Autodesk Inventor part; units mm, degrees
(part 4 of 5)
  line L2655 (4.6359, 9.411) -> (5.6545, 8.2226)
  line L2656 (5.6545, 8.2226) -> (6.2587, 6.9004)
  line L2657 (6.2587, 6.9004) -> (6.4483, 5.4445)
  line L2658 (6.4483, 5.4445) -> (6.2234, 3.8548)
  line L2659 (6.2234, 3.8548) -> (4.7682, 3.4579)
  line L2660 (4.7682, 3.4579) -> (2.8432, 1.5333)
  line L2661 (2.8432, 1.5333) -> (1.064, -0.5108)
  line L2662 (1.064, -0.5108) -> (0.4492, -0.9828)
  line L2663 (0.4492, -0.9828) -> (-0.1305, -1.1181)
  line L2664 (-0.1305, -1.1181) -> (-0.6753, -0.9167)
  line L2665 (-0.6753, -0.9167) -> (-1.185, -0.3785)
  line L2666 (-1.185, -0.3785) -> (-1.2307, 0.9395)
  line L2667 (-1.2307, 0.9395) -> (-1.4443, 2.2167)
  line L2668 (-1.4443, 2.2167) -> (-1.826, 3.453)
  line L2669 (-1.826, 3.453) -> (-2.3756, 4.6485)
  line L2670 (-2.3756, 4.6485) -> (-2.111, 5.31)
  line L2671 (-2.111, 5.31) -> (-2.6223, 7.4795)
  line L2672 (-2.6223, 7.4795) -> (-2.6402, 9.6756)
  line L2673 (-2.6402, 9.6756) -> (-2.036, 11.356)
  line L2674 (-2.036, 11.356) -> (-1.7141, 13.1152)
  line L2675 (-1.7141, 13.1152) -> (0.0057, 15.761)
  line L2676 (-93.9213, 13.6444) -> (-93.19, 13.4597)
  line L2677 (-93.19, 13.4597) -> (-92.7037, 13.0895)
  line L2678 (-92.7037, 13.0895) -> (-92.4624, 12.5337)
  line L2679 (-92.4624, 12.5337) -> (-92.4661, 11.7923)
  line L2680 (-92.4661, 11.7923) -> (-92.7187, 10.8772)
  line L2681 (-92.7187, 10.8772) -> (-93.1336, 10.065)
  line L2682 (-93.1336, 10.065) -> (-93.7109, 9.3558)
  line L2683 (-93.7109, 9.3558) -> (-94.4505, 8.7496)
  line L2684 (-94.4505, 8.7496) -> (-95.0008, 8.6392)
  line L2685 (-95.0008, 8.6392) -> (-95.4488, 8.7347)
  line L2686 (-95.4488, 8.7347) -> (-95.7945, 9.0361)
  line L2687 (-95.7945, 9.0361) -> (-96.038, 9.5433)
  line L2688 (-96.038, 9.5433) -> (-93.9213, 13.6444)
  line L2689 (7.9432, 12.586) -> (8.4146, 12.3444)
  line L2690 (8.4146, 12.3444) -> (8.7702, 11.9992)
  line L2691 (8.7702, 11.9992) -> (9.1338, 10.9985)
  line L2692 (9.1338, 10.9985) -> (9.2661, 10.2048)
  line L2693 (9.2661, 10.2048) -> (9.1338, 9.411)
  line L2694 (9.1338, 9.411) -> (8.6046, 9.1465)
  line L2695 (8.6046, 9.1465) -> (8.0754, 9.411)
  line L2696 (8.0754, 9.411) -> (7.6146, 10.2012)
  line L2697 (7.6146, 10.2012) -> (7.4389, 10.9938)
  line L2698 (7.4389, 10.9938) -> (7.5484, 11.7887)
  line L2699 (7.5484, 11.7887) -> (7.9432, 12.586)
  line L2700 (-111.6484, -1.966) -> (-115.0879, -1.966)
  line L2701 (-115.0879, -1.966) -> (-115.6171, 0.1506)
  line L2702 (-115.6171, 0.1506) -> (-115.0879, 1.4735)
  line L2703 (-115.0879, 1.4735) -> (-115.2202, 6.236)
  line L2704 (-115.2202, 6.236) -> (-116.014, 7.5589)
  line L2705 (-116.014, 7.5589) -> (-116.4749, 9.612)
  line L2706 (-116.4749, 9.612) -> (-117.2046, 11.5277)
  line L2707 (-117.2046, 11.5277) -> (-116.4109, 11.3954)
  line L2708 (-116.4109, 11.3954) -> (-115.3525, 9.8079)
  line L2709 (-115.3525, 9.8079) -> (-114.4461, 9.4186)
  line L2710 (-114.4461, 9.4186) -> (-113.6327, 8.8819)
  line L2711 (-113.6327, 8.8819) -> (-113.3653, 7.6773)
  line L2712 (-113.3653, 7.6773) -> (-112.5744, 6.7652)
  line L2713 (-112.5744, 6.7652) -> (-112.1109, 4.5977)
  line L2714 (-112.1109, 4.5977) -> (-111.802, 2.42)
  line L2715 (-111.802, 2.42) -> (-111.6479, 0.2321)
  line L2716 (-111.6479, 0.2321) -> (-111.6484, -1.966)
  line L2717 (-58.9963, 11.5277) -> (-57.2942, 11.4904)
  line L2718 (-57.2942, 11.4904) -> (-55.6891, 10.9985)
  line L2719 (-55.6891, 10.9985) -> (-55.6883, 9.9418)
  line L2720 (-55.6883, 9.9418) -> (-55.8865, 8.9502)
  line L2721 (-55.8865, 8.9502) -> (-56.2836, 8.0236)
  line L2722 (-56.2836, 8.0236) -> (-56.8797, 7.1621)
  line L2723 (-56.8797, 7.1621) -> (-57.6002, 7.1375)
  line L2724 (-57.6002, 7.1375) -> (-58.2026, 7.5589)
  line L2725 (-58.2026, 7.5589) -> (-58.5305, 7.2355)
  line L2726 (-58.5305, 7.2355) -> (-58.8823, 7.0837)
  line L2727 (-58.8823, 7.0837) -> (-59.258, 7.1033)
  line L2728 (-59.258, 7.1033) -> (-59.6578, 7.2944)
  line L2729 (-59.6578, 7.2944) -> (-59.1319, 9.3325)
  line L2730 (-59.1319, 9.3325) -> (-58.9963, 11.5277)
  line L2731 (-138.1067, 11.2631) -> (-136.4181, 10.9747)
  line L2732 (-136.4181, 10.9747) -> (-134.9317, 10.2048)
  line L2733 (-134.9317, 10.2048) -> (-136.3974, 8.9662)
  line L2734 (-136.3974, 8.9662) -> (-138.1067, 8.0881)
  line L2735 (-138.1067, 8.0881) -> (-138.1067, 11.2631)
  line L2736 (-20.6318, 9.6756) -> (-19.4196, 9.5125)
  line L2737 (-19.4196, 9.5125) -> (-18.2506, 9.1464)
  line L2738 (-18.2506, 9.1464) -> (-18.2905, 7.3941)
  line L2739 (-18.2905, 7.3941) -> (-18.912, 5.7069)
  line L2740 (-18.912, 5.7069) -> (-19.7058, 5.1777)
  line L2741 (-19.7058, 5.1777) -> (-21.2933, 7.2944)
  line L2742 (-21.2933, 7.2944) -> (-21.4336, 8.0061)
  line L2743 (-21.4336, 8.0061) -> (-21.3701, 8.6402)
  line L2744 (-21.3701, 8.6402) -> (-21.1028, 9.1967)
  line L2745 (-21.1028, 9.1967) -> (-20.6318, 9.6756)
  line L2746 (0.7994, 9.1464) -> (1.3625, 9.1738)
  line L2747 (1.3625, 9.1738) -> (1.8148, 9.0286)
  line L2748 (1.8148, 9.0286) -> (2.1563, 8.7108)
  line L2749 (2.1563, 8.7108) -> (2.3869, 8.2204)
  line L2750 (2.3869, 8.2204) -> (2.2879, 7.5492)
  line L2751 (2.2879, 7.5492) -> (2.0565, 7.2152)
  line L2752 (2.0565, 7.2152) -> (1.6926, 7.2184)
  line L2753 (1.6926, 7.2184) -> (1.1963, 7.5589)
  line L2754 (1.1963, 7.5589) -> (0.8732, 8.3219)
  line L2755 (0.8732, 8.3219) -> (0.7994, 9.1464)
  line L2756 (-103.9755, 8.6173) -> (-103.4906, 8.3478)
  line L2757 (-103.4906, 8.3478) -> (-103.2849, 8.0376)
  line L2758 (-103.2849, 8.0376) -> (-103.3583, 7.6864)
  line L2759 (-103.3583, 7.6864) -> (-103.7109, 7.2944)
  line L2760 (-103.7109, 7.2944) -> (-103.9659, 7.9317)
  line L2761 (-103.9659, 7.9317) -> (-103.9755, 8.6173)
  line L2762 (-84.1317, 8.3527) -> (-83.4703, 7.8235)
  line L2763 (-83.4703, 7.8235) -> (-83.341, 6.7532)
  line L2764 (-83.341, 6.7532) -> (-83.6026, 5.7069)
  line L2765 (-83.6026, 5.7069) -> (-84.2653, 6.2709)
  line L2766 (-84.2653, 6.2709) -> (-84.5745, 6.8999)
  line L2767 (-84.5745, 6.8999) -> (-84.53, 7.5938)
  line L2768 (-84.53, 7.5938) -> (-84.1317, 8.3527)
  line L2769 (-29.0985, 7.0298) -> (-28.4104, 6.7294)
  line L2770 (-28.4104, 6.7294) -> (-27.9606, 6.2985)
  line L2771 (-27.9606, 6.2985) -> (-27.749, 5.7372)
  line L2772 (-27.749, 5.7372) -> (-27.7756, 5.0454)
  line L2773 (-27.7756, 5.0454) -> (-28.7088, 5.1098)
  line L2774 (-28.7088, 5.1098) -> (-29.2403, 5.4619)
  line L2775 (-29.2403, 5.4619) -> (-29.3702, 6.1019)
  line L2776 (-29.3702, 6.1019) -> (-29.0985, 7.0298)
  line L2777 (-91.5401, -1.966) -> (-93.3921, -1.966)
  line L2778 (-93.3921, -1.966) -> (-93.2044, -0.9504)
  line L2779 (-93.2044, -0.9504) -> (-92.863, 0.0183)
  line L2780 (-92.863, 0.0183) -> (-93.6713, 0.7264)
  line L2781 (-93.6713, 0.7264) -> (-94.4699, 0.9404)
  line L2782 (-94.4699, 0.9404) -> (-95.2588, 0.6603)
  line L2783 (-95.2588, 0.6603) -> (-96.038, -0.114)
  line L2784 (-96.038, -0.114) -> (-96.5671, -1.966)
  line L2785 (-96.5671, -1.966) -> (-98.9484, -1.966)
  line L2786 (-98.9484, -1.966) -> (-99.3742, -0.3196)
  line L2787 (-99.3742, -0.3196) -> (-100.139, 1.209)
  line L2788 (-100.139, 1.209) -> (-100.8005, 4.6485)
  line L2789 (-100.8005, 4.6485) -> (-100.6806, 5.3724)
  line L2790 (-100.6806, 5.3724) -> (-100.2713, 5.9714)
  line L2791 (-100.2713, 5.9714) -> (-98.1546, 6.7652)
  line L2792 (-98.1546, 6.7652) -> (-97.4932, 6.236)
  line L2793 (-97.4932, 6.236) -> (-97.2526, 5.4664)
  line L2794 (-97.2526, 5.4664) -> (-96.8637, 4.813)
  line L2795 (-96.8637, 4.813) -> (-96.3265, 4.2758)
  line L2796 (-96.3265, 4.2758) -> (-95.6411, 3.8548)
  line L2797 (-95.6411, 3.8548) -> (-95.4814, 3.1188)
  line L2798 (-95.4814, 3.1188) -> (-95.1856, 2.4766)
  line L2799 (-95.1856, 2.4766) -> (-94.7538, 1.9282)
  line L2800 (-94.7538, 1.9282) -> (-94.1859, 1.4735)
  line L2801 (-94.1859, 1.4735) -> (-93.4772, 1.7841)
  line L2802 (-93.4772, 1.7841) -> (-92.863, 2.2673)
  line L2803 (-92.863, 2.2673) -> (-91.9757, 0.2264)
  line L2804 (-91.9757, 0.2264) -> (-91.5401, -1.966)
  line L2805 (16.1452, 6.7652) -> (16.5067, 6.4551)
  line L2806 (16.5067, 6.4551) -> (16.6051, 6.1313)
  line L2807 (16.6051, 6.1313) -> (16.4406, 5.7937)
  line L2808 (16.4406, 5.7937) -> (16.0129, 5.4423)
  line L2809 (16.0129, 5.4423) -> (15.753, 5.7888)
  line L2810 (15.753, 5.7888) -> (15.6885, 6.1249)
  line L2811 (15.6885, 6.1249) -> (15.8192, 6.4503)
  line L2812 (15.8192, 6.4503) -> (16.1452, 6.7652)
  line L2813 (-34.9193, 6.236) -> (-33.5964, 6.236)
  line L2814 (-33.5964, 6.236) -> (-33.6618, 5.6624)
  line L2815 (-33.6618, 5.6624) -> (-33.904, 5.2947)
  line L2816 (-33.904, 5.2947) -> (-34.3232, 5.1331)
  line L2817 (-34.3232, 5.1331) -> (-34.9193, 5.1777)
  line L2818 (-34.9193, 5.1777) -> (-34.9193, 6.236)
  line L2819 (-109.2671, -1.966) -> (-110.0609, -1.966)
  line L2820 (-110.0609, -1.966) -> (-110.4665, 1.5949)
  line L2821 (-110.4665, 1.5949) -> (-110.4577, 5.1777)
  line L2822 (-110.4577, 5.1777) -> (-109.9354, 5.2372)
  line L2823 (-109.9354, 5.2372) -> (-109.5628, 5.0806)
  line L2824 (-109.5628, 5.0806) -> (-109.34, 4.708)
  line L2825 (-109.34, 4.708) -> (-109.2671, 4.1194)
  line L2826 (-109.2671, 4.1194) -> (-109.5755, 2.8028)
  line L2827 (-109.5755, 2.8028) -> (-109.664, 1.4735)
  line L2828 (-109.664, 1.4735) -> (-108.4734, -0.114)
  line L2829 (-108.4734, -0.114) -> (-109.2671, -1.966)
  line L2830 (-138.1067, 4.9131) -> (-137.3778, 4.2285)
  line L2831 (-137.3778, 4.2285) -> (-137.1349, 3.5593)
  line L2832 (-137.1349, 3.5593) -> (-137.3778, 2.9056)
  line L2833 (-137.3778, 2.9056) -> (-138.1067, 2.2673)
  line L2834 (-138.1067, 2.2673) -> (-138.1067, 4.9131)
  line L2835 (-51.588, -1.966) -> (-53.1755, -1.966)
  line L2836 (-53.1755, -1.966) -> (-52.9109, -0.2463)
  line L2837 (-52.9109, -0.2463) -> (-53.9693, 3.8548)
  line L2838 (-53.9693, 3.8548) -> (-53.3078, 4.6485)
  line L2839 (-53.3078, 4.6485) -> (-50.7943, 3.9871)
  line L2840 (-50.7943, 3.9871) -> (-50.3295, 2.8687)
  line L2841 (-50.3295, 2.8687) -> (-50.2651, 1.7381)
  line L2842 (-50.2651, 1.7381) -> (-50.5773, 2.1062)
  line L2843 (-50.5773, 2.1062) -> (-50.8799, 2.2289)
  line L2844 (-50.8799, 2.2289) -> (-51.1727, 2.1062)
  line L2845 (-51.1727, 2.1062) -> (-51.4557, 1.7381)
  line L2846 (-51.4557, 1.7381) -> (-51.3882, -0.1189)
  line L2847 (-51.3882, -0.1189) -> (-51.588, -1.966)
  line L2848 (-98.9484, 4.3839) -> (-98.4586, 4.0963)
  line L2849 (-98.4586, 4.0963) -> (-98.2292, 3.7359)
  line L2850 (-98.2292, 3.7359) -> (-98.2602, 3.3026)
  line L2851 (-98.2602, 3.3026) -> (-98.5515, 2.7965)
  line L2852 (-98.5515, 2.7965) -> (-98.9453, 3.132)
  line L2853 (-98.9453, 3.132) -> (-99.1427, 3.5084)
  line L2854 (-99.1427, 3.5084) -> (-99.1437, 3.9258)
  line L2855 (-99.1437, 3.9258) -> (-98.9484, 4.3839)
  line L2856 (-126.9942, -1.966) -> (-128.0525, -1.966)
  line L2857 (-128.0525, -1.966) -> (-128.5304, 0.1311)
  line L2858 (-128.5304, 0.1311) -> (-128.8463, 2.2673)
  line L2859 (-128.8463, 2.2673) -> (-127.9729, 2.3096)
  line L2860 (-127.9729, 2.3096) -> (-127.1265, 2.5319)
  line L2861 (-127.1265, 2.5319) -> (-126.4825, 2.1569)
  line L2862 (-126.4825, 2.1569) -> (-126.0032, 1.6791)
  line L2863 (-126.0032, 1.6791) -> (-125.6887, 1.0986)
  line L2864 (-125.6887, 1.0986) -> (-125.539, 0.4152)
  line L2865 (-125.539, 0.4152) -> (-126.2062, 0.0071)
  line L2866 (-126.2062, 0.0071) -> (-126.6711, -0.5258)
  line L2867 (-126.6711, -0.5258) -> (-126.9338, -1.1835)
  line L2868 (-126.9338, -1.1835) -> (-126.9942, -1.966)
  line L2869 (-14.2818, -1.966) -> (-15.8693, -1.966)
  line L2870 (-15.8693, -1.966) -> (-15.737, 0.4152)
  line L2871 (-15.737, 0.4152) -> (-14.2818, 2.2673)
  line L2872 (-14.2818, 2.2673) -> (-13.8627, 1.9026)
  line L2873 (-13.8627, 1.9026) -> (-13.7527, 1.3412)
  line L2874 (-13.7527, 1.3412) -> (-14.1743, -0.2873)
  line L2875 (-14.1743, -0.2873) -> (-14.2818, -1.966)
  line L2876 (-127.7879, 2.0027) -> (-127.5418, 1.6552)
  line L2877 (-127.5418, 1.6552) -> (-127.6556, 1.209)
  line L2878 (-127.6556, 1.209) -> (-128.0317, 1.5765)
  line L2879 (-128.0317, 1.5765) -> (-127.7879, 2.0027)
  line L2880 (-118.2629, -1.966) -> (-121.7025, -1.966)
  line L2881 (-121.7025, -1.966) -> (-120.5119, -0.6431)
  line L2882 (-120.5119, -0.6431) -> (-120.0077, 0.6128)
  line L2883 (-120.0077, 0.6128) -> (-119.3213, 1.7381)
  line L2884 (-119.3213, 1.7381) -> (-118.8286, 0.8942)
  line L2885 (-118.8286, 0.8942) -> (-118.488, -0.0044)
  line L2886 (-118.488, -0.0044) -> (-118.2995, -0.9578)
  line L2887 (-118.2995, -0.9578) -> (-118.2629, -1.966)
  line L2888 (15.8806, -1.966) -> (14.8223, -1.966)
  line L2889 (14.8223, -1.966) -> (14.9676, -0.0479)
  line L2890 (14.9676, -0.0479) -> (15.6161, 1.7381)
  line L2891 (15.6161, 1.7381) -> (16.1452, 0.6798)
  line L2892 (16.1452, 0.6798) -> (15.897, -0.6281)
  line L2893 (15.897, -0.6281) -> (15.8806, -1.966)
  line L2894 (-67.9922, 1.4735) -> (-67.6318, 1.2505)
  line L2895 (-67.6318, 1.2505) -> (-67.463, 0.8121)
  line L2896 (-67.463, 0.8121) -> (-67.573, 0.2507)
  line L2897 (-67.573, 0.2507) -> (-67.9922, -0.114)
  line L2898 (-67.9922, -0.114) -> (-68.2291, 0.683)
  line L2899 (-68.2291, 0.683) -> (-67.9922, 1.4735)
  line L2900 (-93.3921, -1.966) -> (-96.5671, -1.966)
  line L2901 (-96.5671, -1.966) -> (-96.038, -0.114)
  line L2902 (-96.038, -0.114) -> (-95.2588, 0.6603)
  line L2903 (-95.2588, 0.6603) -> (-94.4699, 0.9404)
  line L2904 (-94.4699, 0.9404) -> (-93.6713, 0.7264)
  line L2905 (-93.6713, 0.7264) -> (-92.863, 0.0183)
  line L2906 (-92.863, 0.0183) -> (-93.2044, -0.9504)
  line L2907 (-93.2044, -0.9504) -> (-93.3921, -1.966)
  line L2908 (0.0057, -1.966) -> (-1.5818, -1.966)
  line L2909 (-1.5818, -1.966) -> (-1.185, -1.5691)
  line L2910 (-1.185, -1.5691) -> (-0.7881, -1.4368)
  line L2911 (-0.7881, -1.4368) -> (-0.3912, -1.5691)
  line L2912 (-0.3912, -1.5691) -> (0.0057, -1.966)
  point P0 (0, 0)
  constraints: 5826 end point
extrude "Grafika" add sketch "Szkic16" along normal blind 0.6 contours L632 L631 L630 L629 L628 L627 L626 L625 L624 L623 L622 L621 L620 L619 L618 L617 L616 L615 L614 L613 L612 L611 L610 L609 L608 L607 L606 L605 L604 L603 L602 L601 L600 L599 L598 L597 L596 L595 L594 L593 L592 L591 L590 L589 L588 L587 L586 L585 L584 L583 L582 L581 L580 L579 L578 L577 L576 L575 L574 L573 L572 L571 L570 L569 L568 L567 L566 L565 L564 L563 L562 L561 L560 L559 L558 L557 L556 L555 L554 L553 L552 L551 L550 L549 L548 L547 L546 L545 L544 L543 L542 L541 L540 L539 L538 L537 L536 L535 L534 L533 L532 L531 L530 L529 L528 L527 L526 L525 L524 L523 L522 L521 L520 L519 L518 L517 L516 L515 L514 L513 L512 L511 L510 L509 L508 L507 L506 L505 L504 L503 L502 L501 L500 L499 L498 L497 L496 L495 L494 L493 L492 L491 L490 L489 L488 L487 L486 L485 L484 L483 L482 L481 L480 L479 L478 L477 L476 L475 L474 L473 L472 L471 L470 L469 L468 L467 L466 L465 L464 L463 L462 L461 L460 L459 L458 L457 L456 L455 L454 L453 L452 L451 L450 L449 L448 L447 L446 L445 L444 L443 L442 L441 L440 L439 L438 L437 L436 L435 L434 L433 L432 L431 L430 L429 L428 L427 L426 L425 L424 L423 L422 L421 L1458 L1459 L1460 L1461 L1462 L1463 L1464 L1465 L1466 L1467 L1468 L1469 L1470 L1471 L1472 L1473 L1474 L1475 L1476 L1477 L1478 L1479 L1480 L1481 L1482 L1483 L1484 L1485 L1486 L1487 L1488 L1489 L1490 L1491 L1492 L1493 L1494 L1495 L1496 L1497 L1498 L1499 L1500 L1501 L1502 L1503 L1504 L1505 L1506 L1507 L1508 L1509 L1510 L1511 L1512 L1513 L1514 L1515 L1516 L1517 L1518 L1519 L1520 L1521 L1522 L1523 L1524 L1525 L1526 L1527 L1528 L1529 L1530 L1531 L1532 L1533 L1534 L1535 L1536 L1537 L1538 L1539 L1540 L1541 L1542 L1543 L1544 L1545 L1546 L1547 L1548 L1549 L1550 L1551 L1552 L1553 L1554 L1555 L1556 L1557 L1558 L1559 L1560 L1561 L1562 L1563 L1564 L1565 L1566 L1567 L1568 L1569 L1570 L1571 L1572 L1573 L1574 L1575 L1576 L1577 L1578 L1579 L1580 L1581 L1582 L1583 L1584 L1585 L1586 L1587 L1588 | L641 L642 L643 L644 L645 L646 L647 L648 L649 L650 L651 L652 L653 L654 L655 L656 L657 L658 L659 L660 L661 L662 L663 L664 L665 L666 L667 L668 L669 L670 L671 L672 L673 L674 L675 L676 L677 L678 L679 L680 L681 L682 L683 L684 L685 L686 L687 L688 L689 L690 L691 L692 L693 L694 L695 L696 L697 L698 L699 L700 L701 L702 L703 L704 L705 L706 L707 L708 L709 L710 L711 L712 L713 L714 L715 L716 L717 L718 L719 L720 L721 L722 L723 L724 L725 L726 L727 L728 L729 L730 L731 L732 L733 L734 L735 L736 L737 L738 L739 L740 L741 L742 L743 L744 L745 L746 L747 L748 L749 L750 L751 L752 L753 L754 L755 L756 L757 L758 L759 L760 L761 L762 L763 L764 L765 L766 L767 L768 L769 L770 L771 L772 L773 L774 L775 L776 L777 L778 L779 L780 L781 L782 L783 L784 L785 L786 L787 L788 L789 L790 L791 L792 L793 L794 L795 L796 L797 L798 L799 L800 L801 L802 L803 L804 L805 L806 L807 L808 L809 L810 L811 L812 L813 L814 L815 L816 L817 L818 L819 L820 L821 L822 L823 L824 L825 L826 L827 L828 L829 L830 L831 L832 L833 L834 L835 L836 L837 L838 L839 L840 L841 L842 L843 L844 L845 L846 L847 L848 L849 L850 L851 L852 L853 L854 L855 L856 L857 L858 L859 L860 L861 L862 L863 L864 L865 L866 L867 L868 L869 L870 L871 L872 L873 L874 L875 L876 L877 L878 L879 L880 L881 L882 L883 L884 L885 L205 L204 L203 L202 L201 L200 L199 L198 L197 L196 L195 L194 L193 L192 L191 L190 L189 L188 L187 L186 L185 L184 L183 L182 L181 L180 L179 L178 L177 L176 L175 L174 L173 L172 L171 L170 L169 L168 L167 L166 L165 L164 L163 L162 L161 L160 L159 L158 L157 L156 L155 L154 L153 L152 L151 L150 L149 L148 L147 L146 L145 L144 L143 L142 L141 L140 L139 L138 L137 L136 L135 L134 L133 L132 L131 L130 L129 L128 L127 L126 L125 L124 L123 L122 L121 L120 L119 L118 L117 L116 L115 L114 L113 L112 L111 L110 L109 L108 L107 L106 L105 L104 L103 L102 L101 L100 L99 L98 L97 L96 L95 L94 L93 L92 L91 L90 L89 L88 L87 L86 L85 L84 L83 L82 L81 L80 L79 L78 L77 L76 L75 L74 L73 L72 L71 L70 L69 L68 L67 L66 L65 L64 L63 L62 L61 L60 L59 L58 L57 L56 L55 L54 L53 L52 L51 L50 L49 L48 L47 L46 L45 L44 L43 L42 L41 L40 L39 L38 L37 L36 L35 L34 L33 L32 L31 L30 L29 L28 L27 L26 L25 L24 L23 L22 L21 L20 L19 L18 L17 L16 L15 L14 L13 L12 L11 L10 L9 L8 L7 L6 L5 L4 L3 L2 | L1587 L1586 L1585 L1584 L1583 L1582 L1581 L1580 L1579 L1578 L1857 | L1576 L1575 L1574 L1573 L1572 L2134 | L2888 L1153 L1152 L1151 L1150 L1149 | L1570 L1569 L1568 L1567 L1566 L1565 L1564 L2191 | L2908 L826 L825 L824 L823 | L2499 L2498 L2497 L2496 L2495 L2580 | L2869 L2356 L2355 L2354 L2353 L2352 L2351 | L2493 L2492 L2491 L2490 L2735 | L2488 L2487 L2486 L2485 L2834 | L1872 L1873 L1874 L1875 L1876 L1877 L1878 L1879 L1880 L1881 L1882 L1883 L1884 L1885 L1886 L1887 L1888 L1889 L1890 L1891 L1892 L1893 L1894 L1895 L1896 L1897 L1898 L1899 L1900 L1901 L1902 L1903 L1904 L1905 L1906 L1907 L1908 L1909 L1910 L1911 L1912 L1913 L1914 L1915 L1916 L1917 L1918 L1919 L1920 L1921 L1922 L1923 L1924 L391 L390 L389 L388 L387 L386 L385 L384 L383 L382 L381 L380 L379 L378 L377 L376 L375 L374 L373 L372 L371 L370 L369 L368 L367 L366 L365 L364 L363 L362 L361 L360 L359 L358 L357 L356 L355 L354 L353 L352 L351 L350 L349 L348 L347 L346 L345 L344 L343 L342 L341 L340 L339 L338 L337 L336 L335 L334 L333 L332 L331 L330 L329 L328 L327 L326 L325 L324 L323 L322 L321 L320 L319 L318 L317 L316 L315 L314 L313 L312 L311 L310 L309 L308 L307 L306 L305 L304 L303 L302 L301 L300 L299 L298 L297 L296 L295 L294 L293 L292 L291 L290 L289 L288 L287 L286 L285 L284 L283 L282 L281 L280 L279 L278 L277 L276 L275 L274 L273 L272 L271 L270 L269 L268 L267 L266 L265 L264 L263 L262 L261 L260 L259 L258 L257 L256 L255 L254 L253 L252 L251 L250 L249 L248 L247 L246 L245 L244 L243 L242 L241 L240 L239 L238 L237 L236 L235 L234 L233 L232 L231 L230 L229 L228 L227 L226 L225 L224 L223 L222 L221 L220 L219 L218 L217 L216 L215 L214 L213 L212 L211 L210 L209 L208 L207 | L2717 L2718 L2719 L2720 L2721 L2722 L2723 L2724 L2725 L2726 L2727 L2728 L2729 L2730 | L2482 L2481 L2480 L2479 L2478 L2477 L2476 L2475 L2474 L2473 L2472 L2471 L2856 | L2835 L2522 L2521 L2520 L2519 L2518 L2517 L2516 L2515 L2514 L2513 L2512 L2511 | L2622 L419 L418 L417 L416 L415 L414 L413 L412 L411 L410 L409 L408 L407 L406 L405 L404 L403 L402 L401 L400 L399 L398 L397 L396 L395 L394 L393 | L1505 L1504 L1503 L1502 L1501 L1500 L1499 L1498 L1497 L1496 L1495 L1494 L1493 L1492 L1491 L1490 L2700 | L2900 L2784 L2783 L2782 L2781 L2780 L2779 L2778 | L634 L635 L636 L637 L638 L639 L640 | L1090 L1091 L1092 L1093 L1094 L1095 L1096 L1097 | L1098 L1099 L1100 L1101 | L1109 L1110 L1111 L1112 L1113 L1114 L1115 L1116 | L1117 L1118 L1119 L1120 L1121 L1122 L1123 L1124 L1125 L1126 L1127 L1128 L1129 L1130 L1131 | L1132 L1133 L1134 L1135 L1136 L1137 L1138 L1139 L1140 | L1141 L1142 L1143 L1144 L1145 L1146 | L1335 L1336 L1337 L1338 L1339 L1340 | L1341 L1342 L1343 L1344 L1345 L1346 L1347 L1348 L1349 L1350 L1351 L1352 L1353 L1354 L1355 L1356 L1357 L1358 L1359 L1360 L1361 L1362 L1363 L1364 L1365 L1366 L1367 L1368 L1369 | L1370 L1371 L1372 L1373 L1374 L1375 L1376 | L1377 L1378 L1379 L1380 L1381 L1382 L1383 L1384 L1385 L1386 L1387 | L1388 L1389 L1390 L1391 L1392 L1393 L1394 | L1395 L1396 L1397 L1398 L1399 L1400 L1401 L1402 L1403 L1404 L1405 L1406 L1407 L1408 L1409 L1410 L1411 L1412 L1413 L1414 L1415 L1416 L1417 L1418 L1419 L1420 L1421 L1422 L1423 L1424 L1425 L1426 L1427 L1428 L1429 L1430 L1431 L1432 L1433 L1434 L1435 L1436 L1437 L1438 L1439 L1440 L1441 L1442 L1443 L1444 L1445 L1446 L1447 L1448 L1449 | L1801 L1802 L1803 L1804 L1805 L1806 L1807 L1808 L1809 L1810 L1811 L1812 L1813 L1814 L1815 L1816 L1817 L1818 L1819 L1820 L1821 L1822 L1823 L1824 L1825 L1826 L1827 L1828 L1829 L1830 L1831 | L1832 L1833 L1834 L1835 L1836 | L1837 L1838 L1839 L1840 L1841 L1842 L1843 L1844 L1845 L1846 | L1858 L1859 L1860 L1861 | L2121 L2122 L2123 L2124 L2125 L2126 | L2127 L2128 L2129 L2130 L2131 L2132 L2133 | L2140 L2141 L2142 L2143 L2144 L2145 L2146 L2147 L2148 L2149 | L2150 L2151 L2152 L2153 L2154 L2155 L2156 L2157 | L2158 L2159 L2160 L2161 L2162 L2163 L2164 L2165 | L2166 L2167 L2168 L2169 L2170 L2171 | L2172 L2173 L2174 L2175 L2176 L2177 L2178 L2179 | L2180 L2181 L2182 L2183 | L2192 L2193 L2194 L2195 L2196 L2197 L2198 L2199 L2200 L2201 L2202 | L2203 L2204 L2205 L2206 L2207 L2208 L2209 L2210 | L2211 L2212 L2213 L2214 L2215 L2216 L2217 L2218 | L2219 L2220 L2221 L2222 L2223 L2224 L2225 L2226 | L2227 L2228 L2229 L2230 L2231 L2232 L2233 L2234 L2235 L2236 L2237 L2238 L2239 L2240 | L2241 L2242 L2243 L2244 L2245 L2246 L2247 L2248 L2249 | L2250 L2251 L2252 L2253 L2254 L2255 L2256 | L2257 L2258 L2259 L2260 L2261 L2262 | L2263 L2264 L2265 L2266 L2267 L2268 L2269 L2270 L2271 | L2272 L2273 L2274 L2275 L2276 L2277 | L2278 L2279 L2280 | L2298 L2299 L2300 L2301 | L2314 L2315 L2316 L2317 | L2341 L2342 L2343 L2344 L2345 L2346 L2347 L2348 L2349 | L2581 L2582 L2583 L2584 L2585 L2586 | L2594 L2595 L2596 L2597 L2598 | L2605 L2606 L2607 L2608 L2609 L2610 L2611 L2612 L2613 L2614 L2615 L2616 | L2617 L2618 L2619 L2620 L2621 | L2736 L2737 L2738 L2739 L2740 L2741 L2742 L2743 L2744 L2745 | L2746 L2747 L2748 L2749 L2750 L2751 L2752 L2753 L2754 L2755 | L2762 L2763 L2764 L2765 L2766 L2767 L2768 | L2805 L2806 L2807 L2808 L2809 L2810 L2811 L2812 | L2813 L2814 L2815 L2816 L2817 L2818 | L2848 L2849 L2850 L2851 L2852 L2853 L2854 L2855 | L2876 L2877 L2878 L2879
sketch "Szkic11" plane through (0, 45, 0) normal (0, 1, 0) x (1, 0, 0)
  circle A0 centre (-75, 65) radius 4
  line L0 (-3, 100) -> (-107, 100) projected
  line L1 (-55, 100) -> (-55, 0)
  line L2 (-107, 0) -> (-3, 0) projected
  circle A1 centre (-90, 85) radius 4
  circle A2 centre (-75, 32) radius 6.15
  circle A3 centre (-60, 85) radius 4
  line L3 (-110, 97) -> (-110, 3) projected
  line L4 (-110, 97) -> (-110, 100)
  line L5 (-110, 100) -> (-107, 100)
  line L6 (-90, 85) -> (-60, 85)
  line L7 (-32, 85) -> (-12, 85)
  circle A4 centre (-32, 85) radius 3.1
  circle A5 centre (-12, 85) radius 3.1
  line L8 (-42, 69) -> (-22, 69)
  circle A6 centre (-42, 69) radius 3.1
  circle A7 centre (-22, 69) radius 3.1
  line L9 (-75, 85) -> (-75, 65)
  line L10 (-3, 100) -> (-107, 100) projected
  circle A8 centre (-55, 50) radius 2
  point P0 (0, 0)
  point P1 (-55, 100)
  point P2 (-55, 100)
  dimension "d62" = 8
  dimension "d65" = 20
  dimension "d66" = 15
  dimension "d67" = 30
  dimension "d68" = 20
  dimension "d69" = 16
  dimension "d70" = 6.2
  dimension "d71" = 10
  dimension "d72" = 15
  dimension "d73" = 78
  dimension "d74" = 20
  dimension "d104" = 12.3
  dimension "d105" = 35
  dimension "d107" = 68
  dimension "d108" = 4
  dimension "d110" = 55
  dimension "d111" = 50
  constraints: 14 end point, 9 centre point, 5 equal radius, 5 midpoint, 4 coincident, 3 horizontal, 2 vertical, 1 collinear, 1 parallel
  measures "d62" diameter of A1
  measures "d65" horizontal distance of L4.end L6.start
  measures "d66" vertical distance of L4.end L6.start
  measures "d67" distance of L6.end L6.start
  measures "d68" distance of L7.end L7.start
  measures "d69" vertical distance of L8.start L7.start
  measures "d70" diameter of A4
  measures "d71" horizontal distance of L7.start L8.start
  measures "d72" vertical distance of L4.end L7.start
  measures "d73" horizontal distance of L4.end A4.centre
  measures "d74" distance of L9.end L9.start
  measures "d104" diameter of A2
  measures "d105" distance from line of A2.centre L3
  measures "d107" vertical distance of A2.centre point (-55, 100)
  measures "d108" diameter of A8
  measures "d110" distance from line of L3 A8.centre
  measures "d111" distance of point (-55, 100) A8.centre
extrude "Panel" cut sketch "Szkic11" along normal through all both and the other way through all
sketch "Szkic12" plane through (-3, 0, -100) normal (0, 0, -1) x (-1, 0, 0)
  line L0 (0, 0) -> (104, 0) projected
  line L1 (30.3172, 11) -> (39.3172, 11)
  line L2 (39.3172, 11) -> (39.3172, 0)
  line L3 (39.3172, 0) -> (30.3172, 0)
  line L4 (30.3172, 0) -> (30.3172, 11)
  point P0 (-3, 0)
  point P1 (30.3172, 0)
  dimension "d54" = 11
  dimension "d55" = 9
  constraints: 8 end point, 2 parallel, 1 horizontal, 1 perpendicular, 1 point on line
  measures "d54" distance of L3.end L1.start
  measures "d55" distance of L1.start L1.end
extrude "gniazdo DC" cut sketch "Szkic12" against normal up to surface (2 mm away)
sketch "Szkic14" plane through (-102, 43, -98) normal (0, -1, 0) x (1, 0, 0)
  line L0 (95, 22) -> (89, 22)
  line L1 (89, 22) -> (89, 86)
  line L2 (89, 86) -> (95, 86)
  line L3 (95, 86) -> (95, 22)
  circle A0 centre (92, 83) radius 1.2
  circle A1 centre (92, 25) radius 1.2
  line L4 (92, 22) -> (92, 86)
  line L5 (102, 95) -> (102, 1) projected
  line L6 (99, -2) -> (68.6828, -2) projected
  line L7 (95, 22) -> (89, 22)
  line L8 (89, 22) -> (89, 37)
  line L9 (95, 37) -> (95, 22)
  line L10 (95, 86) -> (89, 86)
  line L11 (95, 86) -> (89, 86)
  line L12 (89, 86) -> (89, 68.4398)
  line L13 (95, 76) -> (89, 76)
  line L14 (95, 54) -> (89, 54)
  line L15 (95, 32) -> (89, 32)
  line L16 (46, 22) -> (46, 86)
  line L17 (-3, 22) -> (3, 22)
  line L18 (3, 22) -> (3, 86)
  line L19 (3, 86) -> (-3, 86)
  line L20 (-3, 86) -> (-3, 22)
  circle A2 centre (0, 83) radius 1.2
  circle A3 centre (0, 25) radius 1.2
  line L21 (0, 22) -> (0, 86)
  line L22 (-3, 22) -> (3, 22)
  line L23 (3, 22) -> (3, 37)
  line L24 (-3, 37) -> (-3, 22)
  line L25 (-3, 86) -> (3, 86)
  line L26 (-3, 86) -> (3, 86)
  line L27 (3, 86) -> (3, 68.4398)
  line L28 (-3, 76) -> (3, 76)
  line L29 (-3, 54) -> (3, 54)
  line L30 (-3, 32) -> (3, 32)
  point P0 (102, 98)
  point P1 (3, 76)
  point P2 (3, 32)
  point P3 (-3, 32)
  point P4 (89, 32)
  point P5 (89, 76)
  dimension "d75" = 2.4
  dimension "d76" = 6
  dimension "d77" = 3
  dimension "d78" = 3
  dimension "d79" = 58
  dimension "d91" = 10
  dimension "d92" = 27
  dimension "d98" = 10
  dimension "d99" = 92
  constraints: 58 end point, 22 symmetric about line, 12 point on line, 4 centre point, 4 horizontal, 4 midpoint, 4 perpendicular, 3 parallel, 1 equal radius, 1 vertical, 2 other
  measures "d75" diameter of A1
  measures "d76" distance between parallel lines of L1 L3
  measures "d77" distance from line of L2 A0.centre
  measures "d78" distance from line of L0 A1.centre
  measures "d79" distance of A0.centre A1.centre
  measures "d91" distance from line of L5 A1.centre
  measures "d92" distance from line of L6 A1.centre
  measures "d98" distance between parallel lines of L10 L13
  measures "d99" distance of A3.centre A1.centre
extrude "stelaż PCB" add sketch "Szkic14" along normal blind 35 contours L0 L4 A1 L15 L3 | L0 L1 L15 L4 A1 | L4 A1 | A1 L4 | L13 L4 A0 L2 L3 | L13 L1 L2 L4 A0 | L4 A0 | A0 L4 | L20 L30 L21 A3 L17 | L21 A3 L30 L18 L17 | L21 A3 | A3 L21 | L20 L19 L21 A2 L28 | L21 A2 L19 L18 L28 | L21 A2 | A2 L21
sketch "Szkic15" plane through (-102, 8, -98) normal (0, -1, 0) x (1, 0, 0)
  circle A0 centre (92, 25) radius 1.2 projected
  line L0 (95, 54) -> (89, 54) projected
  line L1 (46, 22) -> (46, 86) projected
  circle A1 centre (92, 25) radius 1.2
  circle A2 centre (92, 83) radius 1.2
  circle A3 centre (0, 25) radius 1.2
  circle A4 centre (0, 83) radius 1.2
  point P0 (102, 98)
  point P1 (92, 83)
  constraints: 4 centre point, 3 symmetric about line, 1 coincident, 1 concentric, 3 other
extrude "inserty stelaz" cut sketch "Szkic15" against normal blind 5.5
sketch "Szkic17" plane through (0, 45, 0) normal (0, 1, 0) x (1, 0, 0)
  line L0 (-110, 97) -> (-110, 3) projected
  line L1 (-42.3172, 100) -> (-107, 100) projected
  line L2 (-3, 100) -> (-33.3172, 100) projected
  line L3 (0, 3) -> (0, 97) projected
  line L4 (-107, 0) -> (-3, 0) projected
  line L5 (-107, 100) -> (-3, 100)
  line L6 (0, 97) -> (0, 3)
  line L7 (-3, 0) -> (-107, 0)
  line L8 (-110, 3) -> (-110, 97)
  line L9 (-3, 100) -> (-107, 100) projected
  line L10 (-110, 97) -> (-110, 53.1539) projected
  line L11 (0, 91.3322) -> (0, 97) projected
  line L12 (-51.3926, 0) -> (-47.7079, 0) projected
  arc A0 (-3, 0) -> (0, 3) centre (-3, 3) ccw
  arc A1 (-110, 3) -> (-107, 0) centre (-107, 3) ccw
  arc A2 (-107, 100) -> (-110, 97) centre (-107, 97) ccw
  arc A3 (0, 97) -> (-3, 100) centre (-3, 97) ccw
  point P0 (0, 0)
  point P1 (-110, 100)
  point P2 (0, 0)
  point P3 (0, 100)
  point P4 (-110, 0)
  dimension "d134" = 3
  dimension "d135" = 3
  constraints: 8 end point, 8 point on circle, 8 point on line, 8 tangent, 4 centre point, 4 collinear, 2 equal radius, 2 parallel, 1 horizontal, 1 perpendicular
  measures "d134" radius of A0
  measures "d135" radius of A1
extrude "bool" cut sketch "Szkic17" along normal mid plane 146.95 keep common part
sketch "Szkic18" plane through (0, 45, 0) normal (0, 1, 0) x (1, 0, 0)
  circle A0 centre (-90, 85) radius 4 projected
  circle A1 centre (-60, 85) radius 4 projected
  circle A2 centre (-75, 65) radius 4 projected
  circle A3 centre (-42, 69) radius 3.1 projected
  circle A4 centre (-32, 85) radius 3.1 projected
  circle A5 centre (-22, 69) radius 3.1 projected
  circle A6 centre (-12, 85) radius 3.1 projected
  arc A7 (-69.3539, 29.5619) -> (-74.5657, 25.8654) centre (-75, 32) ccw projected
  circle A8 centre (-90, 85) radius 4
  circle A9 centre (-60, 85) radius 4 projected
  circle A10 centre (-60, 85) radius 4
  circle A11 centre (-32, 85) radius 3.1
  circle A12 centre (-12, 85) radius 3.1
  circle A13 centre (-22, 69) radius 3.1
  circle A14 centre (-42, 69) radius 3.1
  circle A15 centre (-75, 65) radius 4
  arc A16 (-74.5657, 25.8654) -> (-69.3539, 29.5619) centre (-75, 32) ccw projected
  circle A17 centre (-75, 32) radius 6.15
  circle A18 centre (-90, 85) radius 6
  circle A19 centre (-60, 85) radius 6
  circle A20 centre (-75, 65) radius 6
  circle A21 centre (-42, 69) radius 5.1
  circle A22 centre (-32, 85) radius 5.1
  circle A23 centre (-12, 85) radius 5.1
  circle A24 centre (-22, 69) radius 5.1
  circle A25 centre (-75, 32) radius 8.15
  point P0 (0, 0)
  dimension "obudowa_podkladka_otwory" = 4
  dimension "d116" = 8
  dimension "d117" = 6.2
  dimension "d119" = 12
  dimension "d120" = 12
  dimension "d121" = 12
  dimension "d122" = 10.2
  dimension "d123" = 10.2
  dimension "d124" = 10.2
  dimension "d125" = 10.2
  dimension "d128" = 16.3
  dimension "d129" = 12.3
  constraints: 16 centre point, 16 coincident, 7 concentric
  measures "d116" diameter of A1
  measures "d117" diameter of A11
  measures "d119" diameter of A19
  measures "d120" diameter of A18
  measures "d121" diameter of A20
  measures "d122" diameter of A22
  measures "d123" diameter of A23
  measures "d124" diameter of A21
  measures "d125" diameter of A24
  measures "d128" diameter of A25
  measures "d129" diameter of A17
extrude "Panel_poprawa" add sketch "Szkic18" along normal up to surface (0.6 mm away)
sketch "Szkic19" plane through (0, 45, 0) normal (0, 1, 0) x (1, 0, 0)
  line L0 (-100.9573, 75) -> (-79.0427, 75) construction
  line L1 (-79.0427, 75) -> (-79.0427, 66.8885) construction
  line L2 (-79.0427, 66.8885) -> (-100.9573, 66.8885) construction
  line L3 (-100.9573, 66.8885) -> (-100.9573, 75) construction
  line L4 (-85.9573, 55) -> (-64.0427, 55) construction
  line L5 (-64.0427, 55) -> (-64.0427, 46.8885) construction
  line L6 (-64.0427, 46.8885) -> (-85.9573, 46.8885) construction
  line L7 (-85.9573, 46.8885) -> (-85.9573, 55) construction
  line L8 (-70.9573, 75) -> (-49.0427, 75) construction
  line L9 (-49.0427, 75) -> (-49.0427, 66.8885) construction
  line L10 (-49.0427, 66.8885) -> (-70.9573, 66.8885) construction
  line L11 (-70.9573, 66.8885) -> (-70.9573, 75) construction
  circle A0 centre (-90, 85) radius 4 projected
  line L12 (-90, 85) -> (-90, 75)
  circle A1 centre (-60, 85) radius 4 projected
  line L13 (-60, 85) -> (-60, 75)
  circle A2 centre (-75, 65) radius 4 projected
  line L14 (-75, 65) -> (-75, 55)
  line L15 (-33.0799, 79.9) -> (-33.0799, 90.1) construction
  line L16 (-33.0799, 90.1) -> (-10.9201, 90.1) construction
  line L17 (-10.9201, 90.1) -> (-10.9201, 79.9) construction
  line L18 (-10.9201, 79.9) -> (-33.0799, 79.9) construction
  line L19 (-12.7433, 79.9) -> (-12.7433, 90.1) construction
  line L20 (-12.7433, 90.1) -> (8.7433, 90.1) construction
  line L21 (8.7433, 90.1) -> (8.7433, 79.9) construction
  line L22 (8.7433, 79.9) -> (-12.7433, 79.9) construction
  line L23 (-43.961, 63.9) -> (-43.961, 74.1) construction
  line L24 (-43.961, 74.1) -> (-20.039, 74.1) construction
  line L25 (-20.039, 74.1) -> (-20.039, 63.9) construction
  line L26 (-20.039, 63.9) -> (-43.961, 63.9) construction
  line L27 (-23.4227, 63.9) -> (-23.4227, 74.1) construction
  line L28 (-23.4227, 74.1) -> (-0.5773, 74.1) construction
  line L29 (-0.5773, 74.1) -> (-0.5773, 63.9) construction
  line L30 (-0.5773, 63.9) -> (-23.4227, 63.9) construction
  line L31 (0, 3) -> (0, 15.7523) projected
  circle A3 centre (-32, 85) radius 5.1 projected
  arc A4 (-10.4077, 89.8451) -> (-9.3162, 89.3367) centre (-12, 85) ccw projected
  circle A5 centre (-42, 69) radius 5.1 projected
  circle A6 centre (-22, 69) radius 5.1 projected
  line L32 (-27.1, 59.4066) -> (-27.1, 63) construction
  line L33 (-27.1, 63) -> (-16.9, 63) construction
  line L34 (-16.9, 63) -> (-16.9, 59.4066) construction
  line L35 (-16.9, 59.4066) -> (-27.1, 59.4066) construction
  line L36 (-27.1, 75) -> (-27.1, 78.6821) construction
  line L37 (-27.1, 78.6821) -> (-16.9, 78.6821) construction
  line L38 (-16.9, 78.6821) -> (-16.9, 75) construction
  line L39 (-16.9, 75) -> (-27.1, 75) construction
  line L40 (-47.1, 75) -> (-47.1, 79.3847) construction
  line L41 (-47.1, 79.3847) -> (-36.9, 79.3847) construction
  line L42 (-36.9, 79.3847) -> (-36.9, 75) construction
  line L43 (-36.9, 75) -> (-47.1, 75) construction
  line L44 (-47.1, 59.6228) -> (-47.1, 63) construction
  line L45 (-47.1, 63) -> (-36.9, 63) construction
  line L46 (-36.9, 63) -> (-36.9, 59.6228) construction
  line L47 (-36.9, 59.6228) -> (-47.1, 59.6228) construction
  line L48 (-37.1, 91) -> (-37.1, 94.9889) construction
  line L49 (-37.1, 94.9889) -> (-26.9, 94.9889) construction
  line L50 (-26.9, 94.9889) -> (-26.9, 91) construction
  line L51 (-26.9, 91) -> (-37.1, 91) construction
  line L52 (-17.1, 91) -> (-17.1, 97.0363) construction
  line L53 (-17.1, 97.0363) -> (-6.9, 97.0363) construction
  line L54 (-6.9, 97.0363) -> (-6.9, 91) construction
  line L55 (-6.9, 91) -> (-17.1, 91) construction
  line L56 (-37.1, 76.6304) -> (-37.1, 79) construction
  line L57 (-37.1, 79) -> (-26.9, 79) construction
  line L58 (-26.9, 79) -> (-26.9, 76.6304) construction
  line L59 (-26.9, 76.6304) -> (-37.1, 76.6304) construction
  line L60 (-17.1, 75.8085) -> (-17.1, 79) construction
  line L61 (-17.1, 79) -> (-6.9, 79) construction
  line L62 (-6.9, 79) -> (-6.9, 75.8085) construction
  line L63 (-6.9, 75.8085) -> (-17.1, 75.8085) construction
  line L64 (-96.0049, 75) -> (-94.843, 75)
  line L65 (-94.843, 75) -> (-94.843, 72.6828)
  spline S0 degree 2 poles (-94.843, 72.6828) (-94.843, 72.411) (-94.6683, 72.2298) (-94.4126, 72.2298) knots 0 0 0 1 2 2 2
  line L66 (-94.4126, 72.2298) -> (-94.3511, 72.2298)
  line L67 (-94.3511, 72.2298) -> (-94.3511, 71.0971)
  line L68 (-94.3511, 71.0971) -> (-94.6586, 71.0971)
  spline S1 degree 2 poles (-94.6586, 71.0971) (-95.2961, 71.0971) (-96.0049, 71.8382) (-96.0049, 72.4951) knots 0 0 0 1 2 2 2
  line L69 (-96.0049, 72.4951) -> (-96.0049, 75)
  line L70 (-91.8786, 73.4822) -> (-91.8786, 72.6117)
  line L71 (-91.8786, 72.6117) -> (-92.6359, 72.6117)
  spline S2 degree 2 poles (-92.6359, 72.6117) (-92.7913, 72.6117) (-92.9207, 72.521) (-92.9207, 72.411) knots 0 0 0 1 2 2 2
  spline S3 degree 2 poles (-92.9207, 72.411) (-92.9207, 72.288) (-92.788, 72.2104) (-92.5841, 72.2104) knots 0 0 0 1 2 2 2
  line L72 (-92.5841, 72.2104) -> (-91.8042, 72.2104)
  line L73 (-91.8042, 72.2104) -> (-91.8042, 71.0971)
  line L74 (-91.8042, 71.0971) -> (-92.7168, 71.0971)
  spline S4 degree 2 poles (-92.7168, 71.0971) (-93.3608, 71.0971) (-94.0405, 71.712) (-94.0405, 72.2913) knots 0 0 0 1 2 2 2
  line L75 (-94.0405, 72.2913) -> (-94.0405, 73.822)
  spline S5 degree 2 poles (-94.0405, 73.822) (-94.0405, 74.3819) (-93.3964, 75) (-92.8139, 75) knots 0 0 0 1 2 2 2
  line L76 (-92.8139, 75) -> (-91.8042, 75)
  line L77 (-91.8042, 75) -> (-91.8042, 73.8803)
  line L78 (-91.8042, 73.8803) -> (-92.5453, 73.8803)
  spline S6 degree 2 poles (-92.5453, 73.8803) (-92.8463, 73.8803) (-92.8463, 73.6861) knots 0 0 0 1 1 1
  spline S7 degree 2 poles (-92.8463, 73.6861) (-92.8463, 73.5696) (-92.7039, 73.4822) (-92.5194, 73.4822) knots 0 0 0 1 2 2 2
  line L79 (-92.5194, 73.4822) -> (-91.8786, 73.4822)
  line L80 (-88.3317, 75) -> (-90.034, 70.8738)
  line L81 (-90.034, 70.8738) -> (-91.7233, 75)
  line L82 (-91.7233, 75) -> (-90.3803, 75)
  line L83 (-90.3803, 75) -> (-90.021, 73.7832)
  line L84 (-90.021, 73.7832) -> (-89.6294, 75)
  line L85 (-89.6294, 75) -> (-88.3317, 75)
  line L86 (-85.9984, 73.4822) -> (-85.9984, 72.6117)
  line L87 (-85.9984, 72.6117) -> (-86.7557, 72.6117)
  spline S8 degree 2 poles (-86.7557, 72.6117) (-86.911, 72.6117) (-87.0405, 72.521) (-87.0405, 72.411) knots 0 0 0 1 2 2 2
  spline S9 degree 2 poles (-87.0405, 72.411) (-87.0405, 72.288) (-86.9078, 72.2104) (-86.7039, 72.2104) knots 0 0 0 1 2 2 2
  line L88 (-86.7039, 72.2104) -> (-85.9239, 72.2104)
  line L89 (-85.9239, 72.2104) -> (-85.9239, 71.0971)
  line L90 (-85.9239, 71.0971) -> (-86.8366, 71.0971)
  spline S10 degree 2 poles (-86.8366, 71.0971) (-87.4806, 71.0971) (-88.1602, 71.712) (-88.1602, 72.2913) knots 0 0 0 1 2 2 2
  line L91 (-88.1602, 72.2913) -> (-88.1602, 73.822)
  spline S11 degree 2 poles (-88.1602, 73.822) (-88.1602, 74.3819) (-87.5162, 75) (-86.9337, 75) knots 0 0 0 1 2 2 2
  line L92 (-86.9337, 75) -> (-85.9239, 75)
  line L93 (-85.9239, 75) -> (-85.9239, 73.8803)
  line L94 (-85.9239, 73.8803) -> (-86.665, 73.8803)
  spline S12 degree 2 poles (-86.665, 73.8803) (-86.966, 73.8803) (-86.966, 73.6861) knots 0 0 0 1 1 1
  spline S13 degree 2 poles (-86.966, 73.6861) (-86.966, 73.5696) (-86.8236, 73.4822) (-86.6392, 73.4822) knots 0 0 0 1 2 2 2
  line L95 (-86.6392, 73.4822) -> (-85.9984, 73.4822)
  line L96 (-85.3382, 75) -> (-84.1764, 75)
  line L97 (-84.1764, 75) -> (-84.1764, 72.6828)
  spline S14 degree 2 poles (-84.1764, 72.6828) (-84.1764, 72.411) (-84.0016, 72.2298) (-83.746, 72.2298) knots 0 0 0 1 2 2 2
  line L98 (-83.746, 72.2298) -> (-83.6845, 72.2298)
  line L99 (-83.6845, 72.2298) -> (-83.6845, 71.0971)
  line L100 (-83.6845, 71.0971) -> (-83.9919, 71.0971)
  spline S15 degree 2 poles (-83.9919, 71.0971) (-84.6294, 71.0971) (-85.3382, 71.8382) (-85.3382, 72.4951) knots 0 0 0 1 2 2 2
  line L101 (-85.3382, 72.4951) -> (-85.3382, 75)
  line L102 (-79.178, 53.1877) -> (-78.0744, 53.1877)
  spline S16 degree 2 poles (-78.0744, 53.1877) (-77.7152, 52.7443) (-77.7152, 52.2524) knots 0 0 0 1 1 1
  spline S17 degree 2 poles (-77.7152, 52.2524) (-77.7152, 51.6796) (-78.5534, 50.9029) (-79.165, 50.9029) knots 0 0 0 1 2 2 2
  spline S18 degree 2 poles (-79.165, 50.9029) (-79.9579, 50.9029) (-81.068, 52.11) (-81.068, 52.9773) knots 0 0 0 1 2 2 2
  spline S19 degree 2 poles (-81.068, 52.9773) (-81.068, 53.8447) (-79.9385, 55) (-79.0939, 55) knots 0 0 0 1 2 2 2
  spline S20 degree 2 poles (-79.0939, 55) (-78.8058, 55) (-78.4531, 54.8835) knots 0 0 0 1 1 1
  line L103 (-78.4531, 54.8835) -> (-78.4531, 53.7217)
  spline S21 degree 2 poles (-78.4531, 53.7217) (-78.7282, 53.8511) (-78.9547, 53.8511) knots 0 0 0 1 1 1
  spline S22 degree 2 poles (-78.9547, 53.8511) (-79.3625, 53.8511) (-79.8803, 53.343) (-79.8803, 52.9353) knots 0 0 0 1 2 2 2
  spline S23 degree 2 poles (-79.8803, 52.9353) (-79.8803, 52.521) (-79.4013, 52.0356) (-78.9903, 52.0356) knots 0 0 0 1 2 2 2
  spline S24 degree 2 poles (-78.9903, 52.0356) (-78.7314, 52.0356) (-78.7314, 52.1877) knots 0 0 0 1 1 1
  spline S25 degree 2 poles (-78.7314, 52.1877) (-78.7314, 52.301) (-78.8997, 52.301) knots 0 0 0 1 1 1
  line L104 (-78.8997, 52.301) -> (-79.178, 52.301)
  line L105 (-79.178, 52.301) -> (-79.178, 53.1877)
  line L106 (-75.8285, 52.9579) -> (-75.8285, 51.9288)
  line L107 (-75.8285, 51.9288) -> (-76.1618, 51.9288)
  line L108 (-76.1618, 51.9288) -> (-76.1618, 51)
  line L109 (-76.1618, 51) -> (-77.3236, 51)
  line L110 (-77.3236, 51) -> (-77.3236, 53.4822)
  spline S26 degree 2 poles (-77.3236, 53.4822) (-77.3236, 54.2039) (-76.5372, 55) (-75.8252, 55) knots 0 0 0 1 2 2 2
  spline S27 degree 2 poles (-75.8252, 55) (-75.1392, 55) (-74.4822, 54.2751) (-74.4822, 53.521) knots 0 0 0 1 2 2 2
  line L111 (-74.4822, 53.521) -> (-74.4822, 51)
  line L112 (-74.4822, 51) -> (-75.644, 51)
  line L113 (-75.644, 51) -> (-75.644, 53.4434)
  spline S28 degree 2 poles (-75.644, 53.4434) (-75.644, 53.6731) (-75.7508, 53.8511) (-75.89, 53.8511) knots 0 0 0 1 2 2 2
  spline S29 degree 2 poles (-75.89, 53.8511) (-76.1618, 53.8511) (-76.1618, 53.4434) knots 0 0 0 1 1 1
  line L114 (-76.1618, 53.4434) -> (-76.1618, 52.9579)
  line L115 (-76.1618, 52.9579) -> (-75.8285, 52.9579)
  line L116 (-72.6149, 54.9029) -> (-72.6149, 51)
  line L117 (-72.6149, 51) -> (-73.7767, 51)
  line L118 (-73.7767, 51) -> (-73.7767, 54.9029)
  line L119 (-73.7767, 54.9029) -> (-72.6149, 54.9029)
  line L120 (-71.9159, 51) -> (-71.9159, 53.534)
  spline S30 degree 2 poles (-71.9159, 53.534) (-71.9159, 54.2006) (-71.1165, 55) (-70.4563, 55) knots 0 0 0 1 2 2 2
  spline S31 degree 2 poles (-70.4563, 55) (-69.7929, 55) (-69.0939, 54.2233) (-69.0939, 53.4951) knots 0 0 0 1 2 2 2
  line L121 (-69.0939, 53.4951) -> (-69.0939, 51)
  line L122 (-69.0939, 51) -> (-70.2557, 51)
  line L123 (-70.2557, 51) -> (-70.2557, 53.4951)
  spline S32 degree 2 poles (-70.2557, 53.4951) (-70.2557, 53.8511) (-70.5081, 53.8511) knots 0 0 0 1 1 1
  spline S33 degree 2 poles (-70.5081, 53.8511) (-70.754, 53.8511) (-70.754, 53.4951) knots 0 0 0 1 1 1
  line L124 (-70.754, 53.4951) -> (-70.754, 51)
  line L125 (-70.754, 51) -> (-71.9159, 51)
  line L126 (-64.7573, 73.7832) -> (-64.7573, 71)
  line L127 (-64.7573, 71) -> (-65.9191, 71)
  line L128 (-65.9191, 71) -> (-65.9191, 73.7832)
  line L129 (-65.9191, 73.7832) -> (-66.8091, 73.7832)
  line L130 (-66.8091, 73.7832) -> (-66.8091, 74.9029)
  line L131 (-66.8091, 74.9029) -> (-63.8706, 74.9029)
  line L132 (-63.8706, 74.9029) -> (-63.8706, 73.7832)
  line L133 (-63.8706, 73.7832) -> (-64.7573, 73.7832)
  spline S34 degree 2 poles (-61.5922, 75) (-60.7638, 75) (-59.5793, 73.7929) (-59.5793, 72.9515) knots 0 0 0 1 2 2 2
  spline S35 degree 2 poles (-59.5793, 72.9515) (-59.5793, 72.0971) (-60.7735, 70.9029) (-61.6278, 70.9029) knots 0 0 0 1 2 2 2
  spline S36 degree 2 poles (-61.6278, 70.9029) (-62.4757, 70.9029) (-63.6764, 72.1036) (-63.6764, 72.9515) knots 0 0 0 1 2 2 2
  spline S37 degree 2 poles (-63.6764, 72.9515) (-63.6764, 73.8091) (-62.4693, 75) (-61.5922, 75) knots 0 0 0 1 2 2 2
  spline S38 degree 2 poles (-61.6278, 73.8511) (-61.9838, 73.8511) (-62.4887, 73.3236) (-62.4887, 72.9547) knots 0 0 0 1 2 2 2
  spline S39 degree 2 poles (-62.4887, 72.9547) (-62.4887, 72.5825) (-61.9838, 72.055) (-61.6278, 72.055) knots 0 0 0 1 2 2 2
  spline S40 degree 2 poles (-61.6278, 72.055) (-61.2686, 72.055) (-60.767, 72.5793) (-60.767, 72.9547) knots 0 0 0 1 2 2 2
  spline S41 degree 2 poles (-60.767, 72.9547) (-60.767, 73.3269) (-61.2686, 73.8511) (-61.6278, 73.8511) knots 0 0 0 1 2 2 2
  line L134 (-59.1133, 71) -> (-59.1133, 73.534)
  spline S42 degree 2 poles (-59.1133, 73.534) (-59.1133, 74.2006) (-58.3139, 75) (-57.6537, 75) knots 0 0 0 1 2 2 2
  spline S43 degree 2 poles (-57.6537, 75) (-56.9903, 75) (-56.2913, 74.2233) (-56.2913, 73.4951) knots 0 0 0 1 2 2 2
  line L135 (-56.2913, 73.4951) -> (-56.2913, 71)
  line L136 (-56.2913, 71) -> (-57.4531, 71)
  line L137 (-57.4531, 71) -> (-57.4531, 73.4951)
  spline S44 degree 2 poles (-57.4531, 73.4951) (-57.4531, 73.8511) (-57.7055, 73.8511) knots 0 0 0 1 1 1
  spline S45 degree 2 poles (-57.7055, 73.8511) (-57.9515, 73.8511) (-57.9515, 73.4951) knots 0 0 0 1 1 1
  line L138 (-57.9515, 73.4951) -> (-57.9515, 71)
  line L139 (-57.9515, 71) -> (-59.1133, 71)
  line L140 (-53.5016, 73.3851) -> (-53.5016, 72.5146)
  line L141 (-53.5016, 72.5146) -> (-54.2589, 72.5146)
  spline S46 degree 2 poles (-54.2589, 72.5146) (-54.4142, 72.5146) (-54.5437, 72.4239) (-54.5437, 72.3139) knots 0 0 0 1 2 2 2
  spline S47 degree 2 poles (-54.5437, 72.3139) (-54.5437, 72.1909) (-54.411, 72.1133) (-54.2071, 72.1133) knots 0 0 0 1 2 2 2
  line L142 (-54.2071, 72.1133) -> (-53.4272, 72.1133)
  line L143 (-53.4272, 72.1133) -> (-53.4272, 71)
  line L144 (-53.4272, 71) -> (-54.3398, 71)
  spline S48 degree 2 poles (-54.3398, 71) (-54.9838, 71) (-55.6634, 71.6149) (-55.6634, 72.1942) knots 0 0 0 1 2 2 2
  line L145 (-55.6634, 72.1942) -> (-55.6634, 73.7249)
  spline S49 degree 2 poles (-55.6634, 73.7249) (-55.6634, 74.2848) (-55.0194, 74.9029) (-54.4369, 74.9029) knots 0 0 0 1 2 2 2
  line L146 (-54.4369, 74.9029) -> (-53.4272, 74.9029)
  line L147 (-53.4272, 74.9029) -> (-53.4272, 73.7832)
  line L148 (-53.4272, 73.7832) -> (-54.1683, 73.7832)
  spline S50 degree 2 poles (-54.1683, 73.7832) (-54.4693, 73.7832) (-54.4693, 73.589) knots 0 0 0 1 1 1
  spline S51 degree 2 poles (-54.4693, 73.589) (-54.4693, 73.4725) (-54.3269, 73.3851) (-54.1424, 73.3851) knots 0 0 0 1 2 2 2
  line L149 (-54.1424, 73.3851) -> (-53.5016, 73.3851)
  line L150 (-24.0789, 88.5296) -> (-23.1663, 88.5078)
  spline S52 degree 2 poles (-23.1663, 88.5078) (-23.2561, 87.799) (-24.057, 87.0272) (-24.7002, 87.0272) knots 0 0 0 1 2 2 2
  spline S53 degree 2 poles (-24.7002, 87.0272) (-25.3532, 87.0272) (-26.2342, 87.9034) (-26.2342, 88.5539) knots 0 0 0 1 2 2 2
  spline S54 degree 2 poles (-26.2342, 88.5539) (-26.2342, 89.2068) (-25.3362, 90.1) (-24.6784, 90.1) knots 0 0 0 1 2 2 2
  spline S55 degree 2 poles (-24.6784, 90.1) (-24.0303, 90.1) (-23.5983, 89.6631) knots 0 0 0 1 1 1
  spline S56 degree 2 poles (-23.5983, 89.6631) (-23.2973, 89.3597) (-23.1735, 88.8209) knots 0 0 0 1 1 1
  line L151 (-23.1735, 88.8209) -> (-24.1056, 88.7578)
  spline S57 degree 2 poles (-24.1056, 88.7578) (-24.2633, 89.2383) (-24.7002, 89.2383) knots 0 0 0 1 1 1
  spline S58 degree 2 poles (-24.7002, 89.2383) (-24.9794, 89.2383) (-25.341, 88.8524) (-25.341, 88.5539) knots 0 0 0 1 2 2 2
  spline S59 degree 2 poles (-25.341, 88.5539) (-25.341, 88.2675) (-24.9842, 87.8913) (-24.7124, 87.8913) knots 0 0 0 1 2 2 2
  spline S60 degree 2 poles (-24.7124, 87.8913) (-24.4357, 87.8913) (-24.108, 88.2214) (-24.0789, 88.5296) knots 0 0 0 1 2 2 2
  line L152 (-22.8143, 90.0272) -> (-21.943, 90.0272)
  line L153 (-21.943, 90.0272) -> (-21.943, 88.2893)
  spline S61 degree 2 poles (-21.943, 88.2893) (-21.943, 88.0854) (-21.8119, 87.9495) (-21.6201, 87.9495) knots 0 0 0 1 2 2 2
  line L154 (-21.6201, 87.9495) -> (-21.574, 87.9495)
  line L155 (-21.574, 87.9495) -> (-21.574, 87.1)
  line L156 (-21.574, 87.1) -> (-21.8046, 87.1)
  spline S62 degree 2 poles (-21.8046, 87.1) (-22.2828, 87.1) (-22.8143, 87.6558) (-22.8143, 88.1485) knots 0 0 0 1 2 2 2
  line L157 (-22.8143, 88.1485) -> (-22.8143, 90.0272)
  line L158 (-20.409, 90.0272) -> (-20.409, 87.1)
  line L159 (-20.409, 87.1) -> (-21.2803, 87.1)
  line L160 (-21.2803, 87.1) -> (-21.2803, 90.0272)
  line L161 (-21.2803, 90.0272) -> (-20.409, 90.0272)
  line L162 (-18.8726, 88.1121) -> (-18.8726, 88.8791)
  spline S63 degree 2 poles (-18.8726, 88.8791) (-18.608, 88.8791) (-18.608, 89.0806) knots 0 0 0 1 1 1
  spline S64 degree 2 poles (-18.608, 89.0806) (-18.608, 89.265) (-18.8095, 89.265) knots 0 0 0 1 1 1
  spline S65 degree 2 poles (-18.8095, 89.265) (-19.0133, 89.265) (-19.0133, 89.0126) knots 0 0 0 1 1 1
  line L163 (-19.0133, 89.0126) -> (-19.0133, 87.1)
  line L164 (-19.0133, 87.1) -> (-19.8847, 87.1)
  line L165 (-19.8847, 87.1) -> (-19.8847, 88.9228)
  spline S66 degree 2 poles (-19.8847, 88.9228) (-19.8847, 89.2068) (-19.7706, 89.5684) (-19.6347, 89.7238) knots 0 0 0 1 2 2 2
  spline S67 degree 2 poles (-19.6347, 89.7238) (-19.4794, 89.8985) (-19.0158, 90.1) (-18.7706, 90.1) knots 0 0 0 1 2 2 2
  spline S68 degree 2 poles (-18.7706, 90.1) (-18.324, 90.1) (-17.7172, 89.5005) (-17.7172, 89.0563) knots 0 0 0 1 2 2 2
  spline S69 degree 2 poles (-17.7172, 89.0563) (-17.7172, 88.6243) (-17.9891, 88.3573) knots 0 0 0 1 1 1
  spline S70 degree 2 poles (-17.9891, 88.3573) (-18.2391, 88.1097) (-18.7391, 88.1097) knots 0 0 0 1 1 1
  line L166 (-18.7391, 88.1097) -> (-18.8726, 88.1121)
  line L167 (-15.9405, 74.0272) -> (-15.0692, 74.0272)